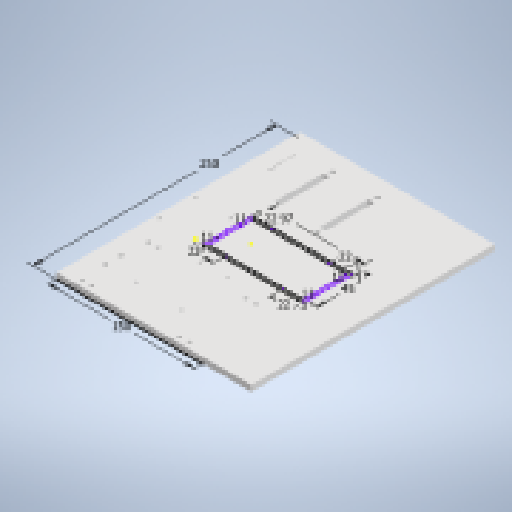
# Autodesk Inventor part: Base
Saved by Autodesk Inventor 2023 (Build 270158000, 158)
## iProperties
Created: 2023-06-06
Part Number: Base
Material: Genérico
Document SubType Name: Modeling
Designer: sergi
Density: 1 g/cm^3
Appearance: Valor por defecto
Author: sergi
Autodesk Inventor part; units mm, degrees
ref_plane "YZ Plane" through (0, 0, 0) normal (1, 0, 0) x (0, 1, 0)
ref_plane "XZ Plane" through (0, 0, 0) normal (0, 1, 0) x (-1, 0, 0)
ref_plane "XY Plane" through (0, 0, 0) normal (0, 0, 1) x (1, 0, 0)
sketch "Boceto1" plane through (0, 0, 0) normal (0, 1, 0) x (-1, 0, 0)
  line L0 (-75, -125) -> (75, -125)
  line L1 (75, -125) -> (75, 125)
  line L2 (75, 125) -> (-75, 125)
  line L3 (-75, 125) -> (-75, -125)
  line L4 (-75, -125) -> (75, 125) construction
  line L5 (75, -125) -> (-75, 125) construction
  point P0 (0, 0)
  dimension "d0" = 150
  dimension "d1" = 250
  constraints: 12 end point, 2 midpoint, 2 parallel, 1 horizontal, 1 perpendicular
  measures "d0" distance of L2.end L1.end
  measures "d1" distance of L0.end L1.end
extrude "Extrusión1" add sketch "Boceto1" along normal blind 6
sketch "Boceto2" plane through (0, 6, 0) normal (0, 1, 0) x (1, 0, 0)
  circle A0 centre (-57, -93) radius 2.3812
  line L0 (-75, -125) -> (75, -125) projected
  line L1 (-75, 125) -> (-75, -125) projected
  circle A1 centre (-57, -77) radius 2.3813
  point P0 (0, 0)
  dimension "d4" = 4.7625
  dimension "d5" = 32
  dimension "d6" = 18
  dimension "d7" = 4.7625
  dimension "d8" = 48
  constraints: 2 centre point
  measures "d4" diameter of A0
  measures "d5" distance from line of L0 A0.centre
  measures "d6" distance from line of L1 A0.centre
  measures "d7" diameter of A1
  measures "d8" distance from line of L0 A1.centre
extrude "Extrusión2" cut sketch "Boceto2" against normal blind 6
sketch "Boceto4" plane through (0, 6, 0) normal (0, 1, 0) x (1, 0, 0)
  circle A0 centre (55, -119) radius 1.9844
  line L0 (75, -125) -> (75, 125) projected
  line L1 (-75, -125) -> (75, -125) projected
  circle A1 centre (45, -119) radius 1.9844
  circle A2 centre (45, -51) radius 1.9844
  circle A3 centre (55, -51) radius 1.9844
  circle A4 centre (-45, -119) radius 1.9844
  circle A5 centre (-45, -51) radius 1.9844
  circle A6 centre (-55, -119) radius 1.9844
  circle A7 centre (-55, -51) radius 1.9844
  line L2 (-75, 125) -> (-75, -125) projected
  line L3 (-26, 50) -> (-20, 50)
  line L4 (-20, 50) -> (-20, 100)
  line L5 (-20, 100) -> (-26, 100)
  line L6 (-26, 100) -> (-26, 50)
  line L7 (75, 125) -> (-75, 125) projected
  line L8 (20, 50) -> (26, 50)
  line L9 (26, 50) -> (26, 100)
  line L10 (26, 100) -> (20, 100)
  line L11 (20, 100) -> (20, 50)
  line L12 (-20, 75) -> (20, 75)
  point P0 (0, 0)
  point P1 (0, 75)
  dimension "d18" = 3.9688
  dimension "d20" = 6
  dimension "d21" = 6
  dimension "d23" = 74
  dimension "d24" = 74
  dimension "d27" = 20
  dimension "d28" = 30
  dimension "d31" = 6
  dimension "d32" = 50
  dimension "d33" = 25
  dimension "d34" = 40
  dimension "d91" = 90
  dimension "d92" = 10
  dimension "d93" = 130
  constraints: 18 end point, 8 centre point, 7 equal radius, 5 horizontal alignment, 4 parallel, 4 vertical alignment, 3 horizontal, 3 midpoint, 2 equal length, 2 perpendicular
  measures "d18" diameter of A0
  measures "d20" distance from line of L1 A0.centre
  measures "d21" distance from line of L1 A1.centre
  measures "d23" distance from line of L1 A3.centre
  measures "d24" distance from line of L1 A2.centre
  measures "d27" distance from line of L2 A6.centre
  measures "d28" distance from line of L2 A4.centre
  measures "d31" distance of L5.end L4.end
  measures "d32" distance of L5.end L3.start
  measures "d33" distance between parallel lines of L7 L5
  measures "d34" distance of L12.start L12.end
  measures "d91" distance of A1.centre A4.centre
  measures "d92" distance of A0.centre A1.centre
  measures "d93" distance from line of L2 A3.centre
extrude "Extrusión3" cut sketch "Boceto4" against normal blind 6 contours A0 | A1 | A2 | A3 | A4 | A5 | A6 | A7 | L6 L5 L4 L3 | L11 L10 L9 L8
sketch "Boceto5" plane through (0, 6, 0) normal (0, 1, 0) x (1, 0, 0)
  line L0 (-59.1058, 74.0163) -> (-59.1058, 128.457) construction
  line L1 (-59.1058, 128.457) -> (-49.5466, 128.457) construction
  line L2 (-49.5466, 128.457) -> (-49.5466, 74.0163) construction
  line L3 (-49.5466, 74.0163) -> (-59.1058, 74.0163) construction
  spline S0 degree 2 poles (-55.8577, 75.3896) (-55.8577, 75.1204) (-55.9985, 74.7202) (-56.1393, 74.5794) knots 0 0 0 1 2 2 2
  spline S1 degree 2 poles (-56.1393, 74.5794) (-56.2973, 74.4189) (-56.7419, 74.288) (-57.068, 74.288) knots 0 0 0 1 2 2 2
  line L4 (-57.068, 74.288) -> (-58.9699, 74.288)
  line L5 (-58.9699, 74.288) -> (-58.9699, 74.6931)
  line L6 (-58.9699, 74.6931) -> (-57.068, 74.6931)
  spline S2 degree 2 poles (-57.068, 74.6931) (-56.8556, 74.6931) (-56.569, 74.7474) (-56.453, 74.824) knots 0 0 0 1 2 2 2
  spline S3 degree 2 poles (-56.453, 74.824) (-56.3295, 74.9055) (-56.2035, 75.1871) (-56.2035, 75.3896) knots 0 0 0 1 2 2 2
  spline S4 degree 2 poles (-56.2035, 75.3896) (-56.2035, 75.5798) (-56.3295, 75.8762) (-56.453, 75.9577) knots 0 0 0 1 2 2 2
  spline S5 degree 2 poles (-56.453, 75.9577) (-56.569, 76.0343) (-56.8531, 76.0886) (-57.0581, 76.0886) knots 0 0 0 1 2 2 2
  line L7 (-57.0581, 76.0886) -> (-58.9699, 76.0886)
  line L8 (-58.9699, 76.0886) -> (-58.9699, 76.4937)
  line L9 (-58.9699, 76.4937) -> (-57.068, 76.4937)
  spline S6 degree 2 poles (-57.068, 76.4937) (-56.7494, 76.4937) (-56.2949, 76.3653) (-56.1393, 76.2022) knots 0 0 0 1 2 2 2
  spline S7 degree 2 poles (-56.1393, 76.2022) (-55.996, 76.0565) (-55.8577, 75.6712) (-55.8577, 75.3896) knots 0 0 0 1 2 2 2
  line L10 (-55.9219, 79.2552) -> (-55.9219, 78.8007)
  line L11 (-55.9219, 78.8007) -> (-58.55, 77.4521)
  line L12 (-58.55, 77.4521) -> (-55.9219, 77.4521)
  line L13 (-55.9219, 77.4521) -> (-55.9219, 77.0742)
  line L14 (-55.9219, 77.0742) -> (-58.9699, 77.0742)
  line L15 (-58.9699, 77.0742) -> (-58.9699, 77.6497)
  line L16 (-58.9699, 77.6497) -> (-56.5567, 78.8773)
  line L17 (-56.5567, 78.8773) -> (-58.9699, 78.8773)
  line L18 (-58.9699, 78.8773) -> (-58.9699, 79.2552)
  line L19 (-58.9699, 79.2552) -> (-55.9219, 79.2552)
  spline S8 degree 2 poles (-55.8676, 81.7697) (-55.8676, 81.5399) (-55.9911, 81.1423) (-56.0602, 81.0114) knots 0 0 0 1 2 2 2
  line L20 (-56.0602, 81.0114) -> (-56.4925, 81.0114)
  line L21 (-56.4925, 81.0114) -> (-56.4925, 81.0311)
  spline S9 degree 2 poles (-56.4925, 81.0311) (-56.453, 81.0805) (-56.3591, 81.2139) (-56.3072, 81.3251) knots 0 0 0 1 2 2 2
  spline S10 degree 2 poles (-56.3072, 81.3251) (-56.2603, 81.4214) (-56.1911, 81.6585) (-56.1911, 81.7845) knots 0 0 0 1 2 2 2
  spline S11 degree 2 poles (-56.1911, 81.7845) (-56.1911, 81.8759) (-56.2331, 82.0858) (-56.2677, 82.1352) knots 0 0 0 1 2 2 2
  spline S12 degree 2 poles (-56.2677, 82.1352) (-56.3146, 82.2069) (-56.4208, 82.2711) (-56.5295, 82.2711) knots 0 0 0 1 2 2 2
  spline S13 degree 2 poles (-56.5295, 82.2711) (-56.6654, 82.2711) (-56.8062, 82.1229) (-56.8531, 81.9327) knots 0 0 0 1 2 2 2
  spline S14 degree 2 poles (-56.8531, 81.9327) (-56.8704, 81.8586) (-56.9198, 81.6215) (-56.947, 81.5202) knots 0 0 0 1 2 2 2
  spline S15 degree 2 poles (-56.947, 81.5202) (-57.0235, 81.2584) (-57.3397, 81.0212) (-57.5645, 81.0212) knots 0 0 0 1 2 2 2
  spline S16 degree 2 poles (-57.5645, 81.0212) (-57.8757, 81.0212) (-58.2635, 81.4881) (-58.2635, 81.8734) knots 0 0 0 1 2 2 2
  spline S17 degree 2 poles (-58.2635, 81.8734) (-58.2635, 82.0636) (-58.1696, 82.4489) (-58.098, 82.5798) knots 0 0 0 1 2 2 2
  line L22 (-58.098, 82.5798) -> (-57.6855, 82.5798)
  line L23 (-57.6855, 82.5798) -> (-57.6855, 82.5601)
  spline S18 degree 2 poles (-57.6855, 82.5601) (-57.8041, 82.4119) (-57.9399, 82.0512) (-57.9399, 81.866) knots 0 0 0 1 2 2 2
  spline S19 degree 2 poles (-57.9399, 81.866) (-57.9399, 81.6758) (-57.7794, 81.414) (-57.6188, 81.414) knots 0 0 0 1 2 2 2
  spline S20 degree 2 poles (-57.6188, 81.414) (-57.4731, 81.414) (-57.3323, 81.5696) (-57.2878, 81.7425) knots 0 0 0 1 2 2 2
  spline S21 degree 2 poles (-57.2878, 81.7425) (-57.2656, 81.8265) (-57.2211, 82.0389) (-57.194, 82.155) knots 0 0 0 1 2 2 2
  spline S22 degree 2 poles (-57.194, 82.155) (-57.1297, 82.4069) (-56.8358, 82.6638) (-56.5814, 82.6638) knots 0 0 0 1 2 2 2
  spline S23 degree 2 poles (-56.5814, 82.6638) (-56.4332, 82.6638) (-56.1714, 82.5477) (-56.075, 82.4341) knots 0 0 0 1 2 2 2
  spline S24 degree 2 poles (-56.075, 82.4341) (-55.9738, 82.3131) (-55.8676, 82.0043) (-55.8676, 81.7697) knots 0 0 0 1 2 2 2
  spline S25 degree 2 poles (-55.87, 84.0149) (-55.87, 83.4666) (-56.4851, 82.8639) (-57.0532, 82.8639) knots 0 0 0 1 2 2 2
  spline S26 degree 2 poles (-57.0532, 82.8639) (-57.6114, 82.8639) (-58.2734, 83.4493) (-58.2734, 83.921) knots 0 0 0 1 2 2 2
  spline S27 degree 2 poles (-58.2734, 83.921) (-58.2734, 84.1335) (-58.1499, 84.462) (-58.0189, 84.583) knots 0 0 0 1 2 2 2
  spline S28 degree 2 poles (-58.0189, 84.583) (-57.888, 84.7065) (-57.5101, 84.8374) (-57.236, 84.8374) knots 0 0 0 1 2 2 2
  line L24 (-57.236, 84.8374) -> (-57.026, 84.8374)
  line L25 (-57.026, 84.8374) -> (-57.026, 83.2541)
  spline S29 degree 2 poles (-57.026, 83.2541) (-56.6283, 83.2541) (-56.206, 83.6543) (-56.206, 84.01) knots 0 0 0 1 2 2 2
  spline S30 degree 2 poles (-56.206, 84.01) (-56.206, 84.1359) (-56.2628, 84.3805) (-56.3072, 84.4793) knots 0 0 0 1 2 2 2
  spline S31 degree 2 poles (-56.3072, 84.4793) (-56.3566, 84.583) (-56.4431, 84.7263) (-56.4826, 84.7732) knots 0 0 0 1 2 2 2
  line L26 (-56.4826, 84.7732) -> (-56.4826, 84.7954)
  line L27 (-56.4826, 84.7954) -> (-56.0627, 84.7954)
  spline S32 degree 2 poles (-56.0627, 84.7954) (-56.0355, 84.7287) (-55.9565, 84.5262) (-55.9343, 84.4472) knots 0 0 0 1 2 2 2
  spline S33 degree 2 poles (-55.9343, 84.4472) (-55.9021, 84.336) (-55.87, 84.1532) (-55.87, 84.0149) knots 0 0 0 1 2 2 2
  spline S34 degree 2 poles (-57.3199, 84.462) (-57.4755, 84.457) (-57.7028, 84.3928) (-57.7794, 84.3311) knots 0 0 0 1 2 2 2
  spline S35 degree 2 poles (-57.7794, 84.3311) (-57.8658, 84.2644) (-57.9572, 84.0544) (-57.9572, 83.8988) knots 0 0 0 1 2 2 2
  spline S36 degree 2 poles (-57.9572, 83.8988) (-57.9572, 83.7457) (-57.8658, 83.5308) (-57.7769, 83.4419) knots 0 0 0 1 2 2 2
  spline S37 degree 2 poles (-57.7769, 83.4419) (-57.6855, 83.3554) (-57.4657, 83.2665) (-57.3199, 83.2541) knots 0 0 0 1 2 2 2
  line L28 (-57.3199, 83.2541) -> (-57.3199, 84.462)
  line L29 (-55.9219, 86.9863) -> (-55.9219, 86.601)
  line L30 (-55.9219, 86.601) -> (-56.1541, 86.601)
  spline S38 degree 2 poles (-56.1541, 86.601) (-56.08, 86.5121) (-55.9812, 86.3812) (-55.9392, 86.2923) knots 0 0 0 1 2 2 2
  spline S39 degree 2 poles (-55.9392, 86.2923) (-55.8997, 86.2107) (-55.8577, 86.0354) (-55.8577, 85.9193) knots 0 0 0 1 2 2 2
  spline S40 degree 2 poles (-55.8577, 85.9193) (-55.8577, 85.7316) (-56.0133, 85.4154) (-56.164, 85.3043) knots 0 0 0 1 2 2 2
  spline S41 degree 2 poles (-56.164, 85.3043) (-56.3146, 85.1931) (-56.7592, 85.0696) (-57.0482, 85.0696) knots 0 0 0 1 2 2 2
  spline S42 degree 2 poles (-57.0482, 85.0696) (-57.3496, 85.0696) (-57.7892, 85.2252) (-57.9547, 85.3611) knots 0 0 0 1 2 2 2
  spline S43 degree 2 poles (-57.9547, 85.3611) (-58.1029, 85.487) (-58.2734, 85.8402) (-58.2734, 86.0354) knots 0 0 0 1 2 2 2
  spline S44 degree 2 poles (-58.2734, 86.0354) (-58.2734, 86.2058) (-58.1968, 86.4602) (-58.1177, 86.601) knots 0 0 0 1 2 2 2
  line L31 (-58.1177, 86.601) -> (-59.1058, 86.601)
  line L32 (-59.1058, 86.601) -> (-59.1058, 86.9863)
  line L33 (-59.1058, 86.9863) -> (-55.9219, 86.9863)
  line L34 (-56.4777, 86.601) -> (-57.7991, 86.601)
  spline S45 degree 2 poles (-57.7991, 86.601) (-57.8683, 86.4577) (-57.9201, 86.2305) (-57.9201, 86.0996) knots 0 0 0 1 2 2 2
  spline S46 degree 2 poles (-57.9201, 86.0996) (-57.9201, 85.8032) (-57.4755, 85.4673) (-57.0556, 85.4673) knots 0 0 0 1 2 2 2
  spline S47 degree 2 poles (-57.0556, 85.4673) (-56.6506, 85.4673) (-56.2232, 85.7242) (-56.2232, 86.0082) knots 0 0 0 1 2 2 2
  spline S48 degree 2 poles (-56.2232, 86.0082) (-56.2232, 86.1589) (-56.3616, 86.4652) (-56.4777, 86.601) knots 0 0 0 1 2 2 2
  spline S49 degree 2 poles (-55.87, 88.5375) (-55.87, 87.9892) (-56.4851, 87.3865) (-57.0532, 87.3865) knots 0 0 0 1 2 2 2
  spline S50 degree 2 poles (-57.0532, 87.3865) (-57.6114, 87.3865) (-58.2734, 87.9719) (-58.2734, 88.4436) knots 0 0 0 1 2 2 2
  spline S51 degree 2 poles (-58.2734, 88.4436) (-58.2734, 88.6561) (-58.1499, 88.9846) (-58.0189, 89.1056) knots 0 0 0 1 2 2 2
  spline S52 degree 2 poles (-58.0189, 89.1056) (-57.888, 89.2291) (-57.5101, 89.36) (-57.236, 89.36) knots 0 0 0 1 2 2 2
  line L35 (-57.236, 89.36) -> (-57.026, 89.36)
  line L36 (-57.026, 89.36) -> (-57.026, 87.7767)
  spline S53 degree 2 poles (-57.026, 87.7767) (-56.6283, 87.7767) (-56.206, 88.1769) (-56.206, 88.5326) knots 0 0 0 1 2 2 2
  spline S54 degree 2 poles (-56.206, 88.5326) (-56.206, 88.6585) (-56.2628, 88.9031) (-56.3072, 89.0019) knots 0 0 0 1 2 2 2
  spline S55 degree 2 poles (-56.3072, 89.0019) (-56.3566, 89.1056) (-56.4431, 89.2489) (-56.4826, 89.2958) knots 0 0 0 1 2 2 2
  line L37 (-56.4826, 89.2958) -> (-56.4826, 89.318)
  line L38 (-56.4826, 89.318) -> (-56.0627, 89.318)
  spline S56 degree 2 poles (-56.0627, 89.318) (-56.0355, 89.2513) (-55.9565, 89.0488) (-55.9343, 88.9698) knots 0 0 0 1 2 2 2
  spline S57 degree 2 poles (-55.9343, 88.9698) (-55.9021, 88.8586) (-55.87, 88.6758) (-55.87, 88.5375) knots 0 0 0 1 2 2 2
  spline S58 degree 2 poles (-57.3199, 88.9846) (-57.4755, 88.9796) (-57.7028, 88.9154) (-57.7794, 88.8537) knots 0 0 0 1 2 2 2
  spline S59 degree 2 poles (-57.7794, 88.8537) (-57.8658, 88.787) (-57.9572, 88.577) (-57.9572, 88.4214) knots 0 0 0 1 2 2 2
  spline S60 degree 2 poles (-57.9572, 88.4214) (-57.9572, 88.2683) (-57.8658, 88.0534) (-57.7769, 87.9645) knots 0 0 0 1 2 2 2
  spline S61 degree 2 poles (-57.7769, 87.9645) (-57.6855, 87.878) (-57.4657, 87.7891) (-57.3199, 87.7767) knots 0 0 0 1 2 2 2
  line L39 (-57.3199, 87.7767) -> (-57.3199, 88.9846)
  line L40 (-55.9219, 92.8551) -> (-55.9219, 91.089)
  line L41 (-55.9219, 91.089) -> (-58.9699, 91.089)
  line L42 (-58.9699, 91.089) -> (-58.9699, 91.4941)
  line L43 (-58.9699, 91.4941) -> (-56.2825, 91.4941)
  line L44 (-56.2825, 91.4941) -> (-56.2825, 92.8551)
  line L45 (-56.2825, 92.8551) -> (-55.9219, 92.8551)
  spline S62 degree 2 poles (-56.164, 94.4186) (-56.1294, 94.3717) (-56.0059, 94.2136) (-55.9688, 94.1395) knots 0 0 0 1 2 2 2
  spline S63 degree 2 poles (-55.9688, 94.1395) (-55.9145, 94.0382) (-55.8577, 93.848) (-55.8577, 93.6751) knots 0 0 0 1 2 2 2
  spline S64 degree 2 poles (-55.8577, 93.6751) (-55.8577, 93.5343) (-55.9639, 93.2799) (-56.0602, 93.1836) knots 0 0 0 1 2 2 2
  spline S65 degree 2 poles (-56.0602, 93.1836) (-56.1541, 93.0922) (-56.4307, 92.9811) (-56.5839, 92.9811) knots 0 0 0 1 2 2 2
  spline S66 degree 2 poles (-56.5839, 92.9811) (-56.821, 92.9811) (-57.1569, 93.1811) (-57.2532, 93.3985) knots 0 0 0 1 2 2 2
  spline S67 degree 2 poles (-57.2532, 93.3985) (-57.3422, 93.5912) (-57.4089, 94.1148) (-57.4261, 94.4186) knots 0 0 0 1 2 2 2
  line L46 (-57.4261, 94.4186) -> (-57.5002, 94.4186)
  spline S68 degree 2 poles (-57.5002, 94.4186) (-57.6336, 94.4186) (-57.7991, 94.3371) (-57.846, 94.263) knots 0 0 0 1 2 2 2
  spline S69 degree 2 poles (-57.846, 94.263) (-57.893, 94.1889) (-57.9226, 93.9765) (-57.9226, 93.8629) knots 0 0 0 1 2 2 2
  spline S70 degree 2 poles (-57.9226, 93.8629) (-57.9226, 93.7295) (-57.8436, 93.3689) (-57.767, 93.1885) knots 0 0 0 1 2 2 2
  line L47 (-57.767, 93.1885) -> (-57.767, 93.1663)
  line L48 (-57.767, 93.1663) -> (-58.1597, 93.1663)
  spline S71 degree 2 poles (-58.1597, 93.1663) (-58.1894, 93.2725) (-58.2635, 93.6702) (-58.2635, 93.8653) knots 0 0 0 1 2 2 2
  spline S72 degree 2 poles (-58.2635, 93.8653) (-58.2635, 94.1024) (-58.1894, 94.426) (-58.093, 94.5545) knots 0 0 0 1 2 2 2
  spline S73 degree 2 poles (-58.093, 94.5545) (-57.9992, 94.6804) (-57.7003, 94.8039) (-57.4854, 94.8039) knots 0 0 0 1 2 2 2
  line L49 (-57.4854, 94.8039) -> (-55.9219, 94.8039)
  line L50 (-55.9219, 94.8039) -> (-55.9219, 94.4186)
  line L51 (-55.9219, 94.4186) -> (-56.164, 94.4186)
  line L52 (-56.4851, 94.4186) -> (-57.1199, 94.4186)
  spline S74 degree 2 poles (-57.1199, 94.4186) (-57.1075, 94.2803) (-57.0655, 93.8629) (-57.026, 93.7319) knots 0 0 0 1 2 2 2
  spline S75 degree 2 poles (-57.026, 93.7319) (-56.9791, 93.5788) (-56.7839, 93.3787) (-56.611, 93.3787) knots 0 0 0 1 2 2 2
  spline S76 degree 2 poles (-56.611, 93.3787) (-56.4134, 93.3787) (-56.2134, 93.601) (-56.2134, 93.8135) knots 0 0 0 1 2 2 2
  spline S77 degree 2 poles (-56.2134, 93.8135) (-56.2134, 93.9938) (-56.369, 94.2902) (-56.4851, 94.4186) knots 0 0 0 1 2 2 2
  spline S78 degree 2 poles (-58.0511, 98.6102) (-57.8535, 98.6102) (-57.4978, 98.4694) (-57.3743, 98.3435) knots 0 0 0 1 2 2 2
  spline S79 degree 2 poles (-57.3743, 98.3435) (-57.2187, 98.1854) (-57.0581, 97.7581) (-57.0581, 97.432) knots 0 0 0 1 2 2 2
  line L53 (-57.0581, 97.432) -> (-57.0581, 97.0887)
  line L54 (-57.0581, 97.0887) -> (-55.9219, 97.0887)
  line L55 (-55.9219, 97.0887) -> (-55.9219, 96.6836)
  line L56 (-55.9219, 96.6836) -> (-58.9699, 96.6836)
  line L57 (-58.9699, 96.6836) -> (-58.9699, 97.4493)
  spline S80 degree 2 poles (-58.9699, 97.4493) (-58.9699, 97.721) (-58.881, 98.1014) (-58.7797, 98.2471) knots 0 0 0 1 2 2 2
  spline S81 degree 2 poles (-58.7797, 98.2471) (-58.6636, 98.4176) (-58.3055, 98.6102) (-58.0511, 98.6102) knots 0 0 0 1 2 2 2
  spline S82 degree 2 poles (-58.0387, 98.1879) (-58.1968, 98.1879) (-58.429, 98.0792) (-58.5031, 97.968) knots 0 0 0 1 2 2 2
  spline S83 degree 2 poles (-58.5031, 97.968) (-58.5673, 97.8717) (-58.6192, 97.6148) (-58.6192, 97.4246) knots 0 0 0 1 2 2 2
  line L58 (-58.6192, 97.4246) -> (-58.6192, 97.0887)
  line L59 (-58.6192, 97.0887) -> (-57.4039, 97.0887)
  line L60 (-57.4039, 97.0887) -> (-57.4039, 97.3653)
  spline S84 degree 2 poles (-57.4039, 97.3653) (-57.4039, 97.6123) (-57.483, 97.9162) (-57.5867, 98.015) knots 0 0 0 1 2 2 2
  spline S85 degree 2 poles (-57.5867, 98.015) (-57.6781, 98.1063) (-57.893, 98.1879) (-58.0387, 98.1879) knots 0 0 0 1 2 2 2
  spline S86 degree 2 poles (-56.164, 100.2404) (-56.1294, 100.1935) (-56.0059, 100.0354) (-55.9688, 99.9613) knots 0 0 0 1 2 2 2
  spline S87 degree 2 poles (-55.9688, 99.9613) (-55.9145, 99.8601) (-55.8577, 99.6699) (-55.8577, 99.497) knots 0 0 0 1 2 2 2
  spline S88 degree 2 poles (-55.8577, 99.497) (-55.8577, 99.3562) (-55.9639, 99.1018) (-56.0602, 99.0054) knots 0 0 0 1 2 2 2
  spline S89 degree 2 poles (-56.0602, 99.0054) (-56.1541, 98.914) (-56.4307, 98.8029) (-56.5839, 98.8029) knots 0 0 0 1 2 2 2
  spline S90 degree 2 poles (-56.5839, 98.8029) (-56.821, 98.8029) (-57.1569, 99.003) (-57.2532, 99.2203) knots 0 0 0 1 2 2 2
  spline S91 degree 2 poles (-57.2532, 99.2203) (-57.3422, 99.413) (-57.4089, 99.9366) (-57.4261, 100.2404) knots 0 0 0 1 2 2 2
  line L61 (-57.4261, 100.2404) -> (-57.5002, 100.2404)
  spline S92 degree 2 poles (-57.5002, 100.2404) (-57.6336, 100.2404) (-57.7991, 100.1589) (-57.846, 100.0848) knots 0 0 0 1 2 2 2
  spline S93 degree 2 poles (-57.846, 100.0848) (-57.893, 100.0107) (-57.9226, 99.7983) (-57.9226, 99.6847) knots 0 0 0 1 2 2 2
  spline S94 degree 2 poles (-57.9226, 99.6847) (-57.9226, 99.5513) (-57.8436, 99.1907) (-57.767, 99.0104) knots 0 0 0 1 2 2 2
  line L62 (-57.767, 99.0104) -> (-57.767, 98.9881)
  line L63 (-57.767, 98.9881) -> (-58.1597, 98.9881)
  spline S95 degree 2 poles (-58.1597, 98.9881) (-58.1894, 99.0944) (-58.2635, 99.492) (-58.2635, 99.6872) knots 0 0 0 1 2 2 2
  spline S96 degree 2 poles (-58.2635, 99.6872) (-58.2635, 99.9243) (-58.1894, 100.2478) (-58.093, 100.3763) knots 0 0 0 1 2 2 2
  spline S97 degree 2 poles (-58.093, 100.3763) (-57.9992, 100.5023) (-57.7003, 100.6258) (-57.4854, 100.6258) knots 0 0 0 1 2 2 2
  line L64 (-57.4854, 100.6258) -> (-55.9219, 100.6258)
  line L65 (-55.9219, 100.6258) -> (-55.9219, 100.2404)
  line L66 (-55.9219, 100.2404) -> (-56.164, 100.2404)
  line L67 (-56.4851, 100.2404) -> (-57.1199, 100.2404)
  spline S98 degree 2 poles (-57.1199, 100.2404) (-57.1075, 100.1021) (-57.0655, 99.6847) (-57.026, 99.5538) knots 0 0 0 1 2 2 2
  spline S99 degree 2 poles (-57.026, 99.5538) (-56.9791, 99.4006) (-56.7839, 99.2006) (-56.611, 99.2006) knots 0 0 0 1 2 2 2
  spline S100 degree 2 poles (-56.611, 99.2006) (-56.4134, 99.2006) (-56.2134, 99.4229) (-56.2134, 99.6353) knots 0 0 0 1 2 2 2
  spline S101 degree 2 poles (-56.2134, 99.6353) (-56.2134, 99.8156) (-56.369, 100.112) (-56.4851, 100.2404) knots 0 0 0 1 2 2 2
  line L68 (-55.9219, 102.6685) -> (-55.9219, 100.9889)
  line L69 (-55.9219, 100.9889) -> (-56.2084, 100.9889)
  line L70 (-56.2084, 100.9889) -> (-57.893, 102.1843)
  line L71 (-57.893, 102.1843) -> (-57.893, 101.0383)
  line L72 (-57.893, 101.0383) -> (-58.2091, 101.0383)
  line L73 (-58.2091, 101.0383) -> (-58.2091, 102.6462)
  line L74 (-58.2091, 102.6462) -> (-57.935, 102.6462)
  line L75 (-57.935, 102.6462) -> (-56.2455, 101.4458)
  line L76 (-56.2455, 101.4458) -> (-56.2455, 102.6685)
  line L77 (-56.2455, 102.6685) -> (-55.9219, 102.6685)
  point P0 (0, 0)
  constraints: 2 other
emboss "Repujado1" sketch "Boceto5" operation cut depth 1 direction (0, -1, 0)
sketch "Boceto6" plane through (0, 6, 0) normal (0, 1, 0) x (1, 0, 0)
  circle A0 centre (23, 44) radius 2.3813
  circle A1 centre (-23, 44) radius 2.3813
  line L0 (-20, 50) -> (-26, 50) projected
  line L1 (26, 50) -> (20, 50) projected
  circle A2 centre (-23, 106) radius 2.3813
  circle A3 centre (23, 106) radius 2.3813
  line L2 (-26, 100) -> (-20, 100) projected
  point P0 (0, 0)
  point P1 (-23, 50)
  point P2 (23, 50)
  point P3 (-23, 50)
  point P4 (-23, 100)
  dimension "d38" = 4.7625
  dimension "d39" = 6
  dimension "d42" = 6
  constraints: 4 centre point, 4 midpoint, 4 vertical alignment, 3 equal radius, 2 horizontal alignment
  measures "d38" diameter of A0
  measures "d39" distance of point (-23, 50) A1.centre
  measures "d42" distance of point (-23, 100) A2.centre
extrude "Extrusión4" cut sketch "Boceto6" against normal through all
sketch "Boceto7" plane through (0, 6, 0) normal (0, 1, 0) x (1, 0, 0)
  circle A0 centre (-10.5, -42.2) radius 1.5
  circle A1 centre (-25.74, -93) radius 1.5
  circle A2 centre (22.52, -94.27) radius 1.5
  circle A3 centre (17.44, -42.2) radius 1.5
  line L0 (-75, -125) -> (75, -125) projected
  line L1 (-75, 125) -> (-75, -125) projected
  point P0 (0, 0)
  dimension "d43" = 3
  dimension "d44" = 82.8
  dimension "d45" = 64.5
  dimension "d46" = 32
  dimension "d47" = 15.24
  dimension "d48" = 27.94
  dimension "d49" = 48.26
  dimension "d50" = 1.27
  constraints: 4 centre point, 3 equal radius, 1 horizontal alignment
  measures "d43" diameter of A0
  measures "d44" distance from line of L0 A0.centre
  measures "d45" distance from line of L1 A0.centre
  measures "d46" distance from line of L0 A1.centre
  measures "d47" horizontal distance of A0.centre A1.centre
  measures "d48" distance of A0.centre A3.centre
  measures "d49" horizontal distance of A1.centre A2.centre
  measures "d50" vertical distance of A2.centre A1.centre
extrude "Extrusión5" cut sketch "Boceto7" against normal through all
sketch "Boceto8" plane through (0, 6, 0) normal (0, 1, 0) x (1, 0, 0)
  circle A0 centre (-70, -24) radius 1.5
  circle A1 centre (-70, 12.5) radius 1.5
  circle A2 centre (-33.5, 12.5) radius 1.5
  circle A3 centre (-33.5, -24) radius 1.5
  line L0 (-75, -125) -> (75, -125) projected
  line L1 (-75, 125) -> (-75, -125) projected
  point P0 (0, 0)
  dimension "d53" = 3
  dimension "d54" = 101
  dimension "d55" = 5
  dimension "d56" = 36.5
  dimension "d57" = 36.5
  constraints: 4 centre point, 3 equal radius, 2 horizontal alignment, 2 vertical alignment
  measures "d53" diameter of A0
  measures "d54" distance from line of L0 A0.centre
  measures "d55" distance from line of L1 A0.centre
  measures "d56" distance of A0.centre A1.centre
  measures "d57" distance of A2.centre A1.centre
extrude "Extrusión6" cut sketch "Boceto8" against normal through all
sketch "Boceto9" plane through (0, 6, 0) normal (0, 1, 0) x (1, 0, 0)
  line L0 (-22, -22.5) -> (75, -22.5)
  line L1 (75, -22.5) -> (75, 22.5)
  line L2 (75, 22.5) -> (-22, 22.5)
  line L3 (-22, 22.5) -> (-22, -22.5)
  line L4 (-25, -25.5) -> (78, -25.5)
  line L5 (78, -25.5) -> (78, 25.5)
  line L6 (78, 25.5) -> (-25, 25.5)
  line L7 (-25, 25.5) -> (-25, -25.5)
  circle A0 centre (-33.5, -24) radius 1.5 projected
  line L8 (-25, -11.5) -> (-22, -11.5)
  line L9 (-22, 11.5) -> (-25, 11.5)
  line L10 (-3, -25.5) -> (-3, -22.5)
  line L11 (56, -25.5) -> (56, -22.5)
  line L12 (-3, 22.5) -> (-3, 25.5)
  line L13 (56, 22.5) -> (56, 25.5)
  line L14 (75, -11.5) -> (78, -11.5)
  line L15 (75, 11.5) -> (78, 11.5)
  point P0 (0, 0)
  point P1 (-25, 0)
  point P2 (-23.5, 11.5)
  point P3 (-3, 24)
  point P4 (76.5, -11.5)
  dimension "d60" = 97
  dimension "d61" = 45
  dimension "d62" = 3
  dimension "d63" = 3
  dimension "d64" = 3
  dimension "d65" = 3
  dimension "d76" = 22
  dimension "d78" = 22
  dimension "d80" = 22
  dimension "d81" = 22
  dimension "d84" = 11
  dimension "d86" = 11
  dimension "d87" = 11
  dimension "d88" = 11
  constraints: 32 end point, 16 point on line, 7 perpendicular, 5 parallel, 4 midpoint, 3 horizontal, 1 horizontal alignment, 1 vertical
  measures "d60" distance of L1.end L2.end
  measures "d61" distance of L0.end L1.end
  measures "d62" distance between parallel lines of L5 L1
  measures "d63" distance between parallel lines of L6 L2
  measures "d64" distance between parallel lines of L4 L0
  measures "d65" distance between parallel lines of L7 L3
  measures "d76" distance between parallel lines of L5 L11
  measures "d78" distance between parallel lines of L5 L13
  measures "d80" distance between parallel lines of L7 L10
  measures "d81" distance from line of L7 point (-3, 24)
  measures "d84" distance between parallel lines of L8 L0
  measures "d86" distance between parallel lines of L2 L9
  measures "d87" distance from line of point (76.5, -11.5) L0
  measures "d88" distance between parallel lines of L2 L15
sketch "Boceto12" plane through (75, 0, 125) normal (1, 0, 0) x (0, 0, -1)
  line L0 (0, 0) -> (0, 6) projected
  line L1 (250, 0) -> (250, 6) projected
  line L2 (0, 6) -> (250, 6)
  line L3 (250, 6) -> (250, 0)
  line L4 (250, 0) -> (0, 0)
  line L5 (0, 0) -> (0, 6)
  point P0 (125, 0)
  constraints: 8 end point, 2 parallel, 1 horizontal, 1 perpendicular
